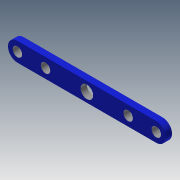
# Autodesk Inventor part: tahlo4(2)
Saved by Autodesk Inventor 2013 (Build 170138000, 138)
## iProperties
Created: 2013-02-03
Part Number: tahlo4(2)
Material: Generic
Document SubType Name: Modeling
Designer: idle-rug
Density: 1 g/cm^3
Author: idle-rug
Autodesk Inventor part; units mm, degrees
ref_plane "YZ Plane" through (0, 0, 0) normal (1, 0, 0) x (0, 1, 0)
ref_plane "XZ Plane" through (0, 0, 0) normal (0, 1, 0) x (-1, 0, 0)
ref_plane "XY Plane" through (0, 0, 0) normal (0, 0, 1) x (1, 0, 0)
sketch "Sketch1" plane through (0, 0, 0) normal (0, 1, 0) x (-1, 0, 0)
  line L0 (22, 3) -> (-22, 3)
  line L1 (-22, 3) -> (-22, -3)
  line L2 (-22, -3) -> (22, -3)
  line L3 (22, -3) -> (22, 3)
  line L4 (22, 3) -> (-22, -3) construction
  line L5 (-22, 3) -> (22, -3) construction
  circle A0 centre (-22, 0) radius 3
  circle A1 centre (22, 0) radius 3
  point P0 (0, 0)
  dimension "d0" = 44
  dimension "d1" = 6
  dimension "d2" = 6
  dimension "d3" = 6
  constraints: 12 end point, 4 midpoint, 2 centre point, 2 parallel, 1 horizontal, 1 perpendicular
  measures "d0" distance of L2.end L1.end
  measures "d1" distance of L1.end L0.end
  measures "d2" diameter of A0
  measures "d3" diameter of A1
extrude "Extrusion1" add sketch "Sketch1" along normal blind 2
sketch "Sketch2" plane through (0, 2, 0) normal (0, 1, 0) x (1, 0, 0)
  arc A0 (-22, 3) -> (-22, -3) centre (-22, 0) ccw projected
  arc A1 (22, -3) -> (22, 3) centre (22, 0) ccw projected
  circle A2 centre (-22, 0) radius 1.5
  circle A3 centre (0, 0) radius 1.5
  circle A4 centre (22, 0) radius 1.5
  dimension "d6" = 3
  dimension "d7" = 3
  dimension "d8" = 3
  constraints: 3 centre point, 3 coincident
  measures "d6" diameter of A2
  measures "d7" diameter of A3
  measures "d8" diameter of A4
extrude "Extrusion2" cut sketch "Sketch2" against normal blind 2
sketch "Sketch3" plane through (0, 0, 0) normal (0, -1, 0) x (1, 0, 0)
  circle A0 centre (0, 0) radius 1.5 projected
  line L0 (22, -3) -> (-22, -3) projected
  line L1 (0, 0) -> (-10, 0)
  circle A1 centre (-10, 0) radius 1.5
  dimension "d11" = 10
  dimension "d12" = 3
  constraints: 2 end point, 1 centre point, 1 coincident, 1 parallel
  measures "d11" distance of L1.start L1.end
  measures "d12" diameter of A1
extrude "Extrusion3" cut sketch "Sketch3" against normal blind 2 contours A1
sketch "Sketch4" plane through (0, 0, 0) normal (0, -1, 0) x (1, 0, 0)
  circle A0 centre (-10, 0) radius 1.5 projected
  circle A1 centre (0, 0) radius 1.5 projected
  circle A2 centre (-22, 0) radius 1.5 projected
  arc A3 (-22, 3) -> (-22, -3) centre (-22, 0) ccw projected
  arc A4 (22, -3) -> (22, 3) centre (22, 0) ccw projected
  circle A5 centre (-22, 0) radius 0.1
  circle A6 centre (-10, 0) radius 0.1
  circle A7 centre (0, 0) radius 0.1
  circle A8 centre (22, 0) radius 0.1
  dimension "d15" = 0.2
  dimension "d16" = 0.2
  dimension "d17" = 0.2
  dimension "d18" = 0.2
  constraints: 4 centre point, 4 coincident
  measures "d15" diameter of A5
  measures "d16" diameter of A6
  measures "d17" diameter of A7
  measures "d18" diameter of A8
extrude "Extrusion4" add sketch "Sketch4" against normal blind 2 contours A0 | A1 | A2
sketch "Sketch5" plane through (0, 0, 0) normal (0, -1, 0) x (1, 0, 0)
  circle A0 centre (22, 0) radius 1.5 projected
  arc A1 (22, -3) -> (22, 3) centre (22, 0) ccw projected
  circle A2 centre (22, 0) radius 0.1
  dimension "d21" = 0.2
  constraints: 1 centre point, 1 coincident
  measures "d21" diameter of A2
extrude "Extrusion5" add sketch "Sketch5" against normal blind 2
sketch "Sketch6" plane through (0, 2, 0) normal (0, 1, 0) x (1, 0, 0)
  circle A0 centre (0, 0) radius 0.1 projected
  line L0 (-22, -3) -> (22, -3) projected
  line L1 (0, 0) -> (-12.985, 0)
  circle A1 centre (-12.985, 0) radius 0.1
  line L2 (0, 0) -> (12.985, 0)
  circle A2 centre (12.985, 0) radius 0.1
  dimension "d24" = 12.985
  dimension "d25" = 0.2
  dimension "d26" = 12.985
  dimension "d27" = 0.2
  constraints: 4 end point, 2 centre point, 2 coincident, 1 collinear, 1 parallel
  measures "d24" distance of L1.start L1.end
  measures "d25" diameter of A1
  measures "d26" distance of L1.start L2.end
  measures "d27" diameter of A2
extrude "Extrusion6" cut sketch "Sketch6" against normal blind 2 contours A1 | A2
sketch "Sketch7" plane through (0, 2, 0) normal (0, 1, 0) x (1, 0, 0)
  circle A0 centre (-10, 0) radius 0.1 projected
extrude "Extrusion7" add sketch "Sketch7" against normal blind 2
sketch "Sketch8" plane through (0, 2, 0) normal (0, 1, 0) x (1, 0, 0)
  circle A0 centre (-12.985, 0) radius 0.1 projected
  circle A1 centre (12.985, 0) radius 0.1 projected
extrude "Extrusion8" add sketch "Sketch8" against normal blind 2
sketch "Sketch9" plane through (0, 2, 0) normal (0, 1, 0) x (1, 0, 0)
  circle A0 centre (-13.093, 0) radius 0.1
  circle A1 centre (13.093, 0) radius 0.1
  dimension "d35" = 0.2
  dimension "d36" = 0.2
  constraints: 2 centre point
  measures "d35" diameter of A0
  measures "d36" diameter of A1
extrude "Extrusion9" cut sketch "Sketch9" against normal blind 2
extrude "Extrusion10" [suppressed]
sketch "Sketch11" plane through (0, 2, 0) normal (0, 1, 0) x (1, 0, 0)
  circle A0 centre (0, 0) radius 2 projected
  circle A1 centre (13.093, 0) radius 1.5 projected
  circle A2 centre (-13.093, 0) radius 1.5 projected
  circle A3 centre (-22, 0) radius 1.5 projected
  circle A4 centre (22, 0) radius 1.5 projected
extrude "Extrusion11" cut sketch "Sketch11" against normal blind 2
body "Solid1"
